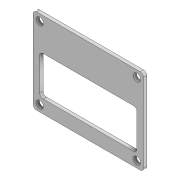
# Autodesk Inventor part: cosmic-watch-endplate
Saved by Autodesk Inventor 2020 (Build 240168000, 168)
## iProperties
Created: 2020-03-05
Part Number: cosmic-watch-endplate
Material: Generic
Document SubType Name: Modeling
Designer: kaduo
Density: 1 g/cm^3
Appearance: Default
Author: kaduo
Autodesk Inventor part; units mm, degrees
ref_plane "YZ Plane" through (0, 0, 0) normal (1, 0, 0) x (0, 1, 0)
ref_plane "XZ Plane" through (0, 0, 0) normal (0, 1, 0) x (-1, 0, 0)
ref_plane "XY Plane" through (0, 0, 0) normal (0, 0, 1) x (1, 0, 0)
sketch "Sketch1" plane through (0, 0, 0) normal (0, 0, 1) x (1, 0, 0)
  line L0 (0, 0) -> (67.31, 0)
  line L1 (67.31, 0) -> (67.31, 52)
  line L2 (67.31, 52) -> (0, 52)
  line L3 (0, 52) -> (0, 0)
  line L4 (4, 8) -> (63.31, 8)
  line L5 (63.31, 8) -> (63.31, 32)
  line L6 (63.31, 32) -> (4, 32)
  line L7 (4, 32) -> (4, 8)
  dimension "d0" = 67.31
  dimension "d1" = 52
  dimension "d2" = 59.31
  dimension "d4" = 4
  dimension "d5" = 8
  dimension "d19" = 20
  constraints: 16 end point, 4 parallel, 2 horizontal, 2 perpendicular
  measures "d0" distance of L2.end L1.end
  measures "d1" distance of L1.end L0.end
  measures "d2" distance of L6.end L5.end
  measures "d4" distance between parallel lines of L3 L7
  measures "d5" distance between parallel lines of L0 L4
  measures "d19" distance between parallel lines of L6 L2
extrude "Extrusion1" add sketch "Sketch1" along normal blind 2
sketch "Sketch2" plane through (0, 0, 2) normal (0, 0, 1) x (1, 0, 0)
  line L0 (0, 0) -> (67.31, 0) projected
  line L1 (4, 0) -> (4, 39.8865)
  line L2 (0, 52) -> (0, 0) projected
  line L3 (0, 48) -> (67.31, 48)
  line L4 (63.31, 39.878) -> (63.31, 0)
  line L5 (0, 4) -> (67.31, 4)
  line L6 (67.31, 52) -> (0, 52) projected
  line L7 (67.31, 0) -> (67.31, 52) projected
  point P0 (4, 48)
  point P1 (4, 4)
  point P2 (63.31, 4)
  point P3 (63.31, 48)
  dimension "d8" = 4
  dimension "d9" = 4
  dimension "d10" = 4
  dimension "d11" = 4
  constraints: 12 point on line, 8 end point, 3 perpendicular, 1 vertical, 1 other
  measures "d8" distance between parallel lines of L2 L1
  measures "d10" distance between parallel lines of L7 L4
  measures "d11" distance between parallel lines of L0 L5
hole "Hole1" at (4, 48, 2) at (4, 4, 2) at (63.31, 4, 2) at (63.31, 48, 2) direction (0, 0, -1) diameter 4.5 end through all
fillet "Fillet1" radius 2 4 edges at (0, 52, 1) (0, 0, 1) (67.31, 0, 1) (67.31, 52, 1)
fillet "Fillet2" radius 2 4 edges at (63.31, 8, 1) (63.31, 32, 1) (4, 32, 1) (4, 8, 1)
body "Solid1"
